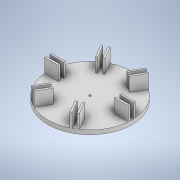
# Autodesk Inventor part: outer_hub
Saved by Autodesk Inventor 2020 (Build 240168000, 168)
## iProperties
Created: 2019-09-24
Part Number: outer_hub
Material: Generic
Document SubType Name: Modeling
Designer: dlr6513
Density: 1 g/cm^3
Appearance: Default
Author: dlr6513
Autodesk Inventor part; units mm, degrees
ref_plane "YZ Plane" through (0, 0, 0) normal (1, 0, 0) x (0, 1, 0)
ref_plane "XZ Plane" through (0, 0, 0) normal (0, 1, 0) x (-1, 0, 0)
ref_plane "XY Plane" through (0, 0, 0) normal (0, 0, 1) x (1, 0, 0)
sketch "Sketch1" plane through (0, 0, 0) normal (0, 1, 0) x (-1, 0, 0)
  circle A0 centre (0, 0) radius 60
  circle A1 centre (0, 0) radius 1.5
  line L0 (40, -2.5) -> (40, -5)
  line L1 (40, -5) -> (59.7913, -5)
  line L2 (40, 2.5) -> (40, 5)
  line L3 (40, 5) -> (59.7913, 5)
  line L4 (40, -2.5) -> (59.9479, -2.5)
  line L5 (40, 2.5) -> (59.9479, 2.5)
  line L6 (15.6699, 37.141) -> (25.5655, 54.2808)
  line L7 (17.8349, 35.891) -> (27.8089, 53.1664)
  line L8 (17.8349, 35.891) -> (15.6699, 37.141)
  line L9 (22.1651, 33.391) -> (32.139, 50.6664)
  line L10 (24.3301, 32.141) -> (34.2258, 49.2808)
  line L11 (22.1651, 33.391) -> (24.3301, 32.141)
  line L12 (-24.3301, 32.141) -> (-34.2258, 49.2808)
  line L13 (-22.1651, 33.391) -> (-32.139, 50.6664)
  line L14 (-22.1651, 33.391) -> (-24.3301, 32.141)
  line L15 (-17.8349, 35.891) -> (-27.8089, 53.1664)
  line L16 (-15.6699, 37.141) -> (-25.5655, 54.2808)
  line L17 (-17.8349, 35.891) -> (-15.6699, 37.141)
  line L18 (-40, -5) -> (-59.7913, -5)
  line L19 (-40, -2.5) -> (-59.9479, -2.5)
  line L20 (-40, -2.5) -> (-40, -5)
  line L21 (-40, 2.5) -> (-59.9479, 2.5)
  line L22 (-40, 5) -> (-59.7913, 5)
  line L23 (-40, 2.5) -> (-40, 5)
  line L24 (-15.6699, -37.141) -> (-25.5655, -54.2808)
  line L25 (-17.8349, -35.891) -> (-27.8089, -53.1664)
  line L26 (-17.8349, -35.891) -> (-15.6699, -37.141)
  line L27 (-22.1651, -33.391) -> (-32.139, -50.6664)
  line L28 (-24.3301, -32.141) -> (-34.2258, -49.2808)
  line L29 (-22.1651, -33.391) -> (-24.3301, -32.141)
  line L30 (24.3301, -32.141) -> (34.2258, -49.2808)
  line L31 (22.1651, -33.391) -> (32.139, -50.6664)
  line L32 (22.1651, -33.391) -> (24.3301, -32.141)
  line L33 (17.8349, -35.891) -> (27.8089, -53.1664)
  line L34 (15.6699, -37.141) -> (25.5655, -54.2808)
  line L35 (17.8349, -35.891) -> (15.6699, -37.141)
  point P0 (60, -5)
  point P1 (60, 5)
  point P2 (60, -2.5)
  point P3 (60, 2.5)
  dimension "d0" = 120
  dimension "d1" = 3
  dimension "d8" = 360
  constraints: 72 end point, 4 point on circle, 2 centre point, 2 coincident, 85 other
  measures "d0" diameter of A0
  measures "d1" diameter of A1
extrude "Extrusion1" add sketch "Sketch1" along normal blind 6 contours A0 L4 L0 L1 L30 L32 L31 L33 L35 L34 L24 L26 L25 L27 L29 L28 L18 L20 L19 L21 L23 L22 L12 L14 L13 L15 L17 L16 L6 L8 L7 L9 L11 L10 L3 L2 L5
extrude "Extrusion2" add sketch "Sketch1" along normal blind 26 contours L5 L2 L3 A0 | A0 L1 L0 L4 | L10 L11 L9 A0 | A0 L31 L32 L30 | L7 L8 L6 A0 | A0 L34 L35 L33 | L16 L17 L15 A0 | A0 L25 L26 L24 | L13 L14 L12 A0 | A0 L28 L29 L27 | L22 L23 L21 A0 | A0 L19 L20 L18
body "Solid1"
